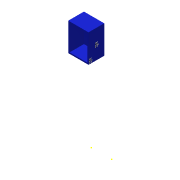
# Autodesk Inventor part: Bucket blue
Saved by Autodesk Inventor 2015 (Build 190159000, 159)
## iProperties
Created: 2015-04-10
Part Number: Bucket blue
Material: Generic
Document SubType Name: Modeling
Designer: Vukica
Density: 1 g/cm^3
Appearance: Blue - Wall Paint - Glossy
Author: Vukica
Autodesk Inventor part; units mm, degrees
ref_plane "YZ Plane" through (0, 0, 0) normal (1, 0, 0) x (0, 1, 0)
ref_plane "XZ Plane" through (0, 0, 0) normal (0, 1, 0) x (-1, 0, 0)
ref_plane "Work Plane1" through (220.5144, 586.5816, 98.3522) normal (0, 0, 1) x (1, 0, 0)
sketch "Sketch1" plane through (220.5144, 586.5816, 98.3522) normal (0, 0, 1) x (1, 0, 0)
  line L0 (12.7, 622.3) -> (215.9, 622.3)
  line L1 (12.7, 317.5) -> (215.9, 317.5)
  line L2 (241.3, 317.5) -> (241.3, 596.9)
  line L3 (-12.7, 596.9) -> (-12.7, 317.5)
  line L4 (215.9, 596.9) -> (12.7, 596.9)
  line L5 (215.9, 596.9) -> (215.9, 317.5)
  line L6 (12.7, 317.5) -> (12.7, 596.9)
  line L7 (212.725, 593.725) -> (15.875, 593.725)
  line L8 (15.875, 593.725) -> (15.875, 320.675)
  line L9 (15.875, 320.675) -> (212.725, 320.675)
  line L10 (212.725, 320.675) -> (212.725, 593.725)
  point P0 (-220.5144, -586.5816)
extrude "Extrusion1" add sketch "Sketch1" along normal blind 127 and the other way blind 25.4 contours L10 L9 L8 L7
shell "Shell1" thickness 12.7 removed faces 1 at (302.006, 1089.2899, 225.3522)
sketch "Sketch2" plane through (433.2394, 907.2566, 225.3522) normal (1, 0, 0) x (0, 0, -1)
  line L0 (3.6537, 3.0906) -> (3.6537, 49.4858) construction
  line L1 (3.6537, 49.4858) -> (36.2785, 49.4858) construction
  line L2 (36.2785, 49.4858) -> (36.2785, 3.0906) construction
  line L3 (36.2785, 3.0906) -> (3.6537, 3.0906) construction
  line L4 (64.1536, 108.921) -> (64.1536, 155.3161) construction
  line L5 (64.1536, 155.3161) -> (96.7784, 155.3161) construction
  line L6 (96.7784, 155.3161) -> (96.7784, 108.921) construction
  line L7 (96.7784, 108.921) -> (64.1536, 108.921) construction
  point P0 (225.3522, -907.2566)
  constraints: 4 other
sketch "Sketch3" plane through (236.3894, 907.2566, 225.3522) normal (-1, 0, 0) x (0, 0, 1)
  line L0 (-64.8568, 166.6409) -> (-64.8568, 120.2457) construction
  line L1 (-64.8568, 120.2457) -> (-97.4816, 120.2457) construction
  line L2 (-97.4816, 120.2457) -> (-97.4816, 166.6409) construction
  line L3 (-97.4816, 166.6409) -> (-64.8568, 166.6409) construction
  line L4 (-4.4124, 269.0962) -> (-4.4124, 222.701) construction
  line L5 (-4.4124, 222.701) -> (-37.0372, 222.701) construction
  line L6 (-37.0372, 222.701) -> (-37.0372, 269.0962) construction
  line L7 (-37.0372, 269.0962) -> (-4.4124, 269.0962) construction
  point P0 (-225.3522, -907.2566)
  constraints: 4 other
body "Solid1"
